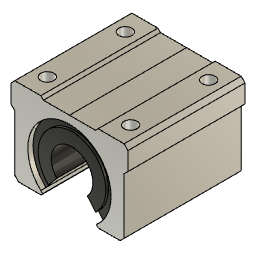
SBR16UU (Autodesk Fusion 360 design; units mm, degrees)
Autodesk Fusion 360 part; units mm, degrees
sketch "Front" plane through (0, 0, 0) normal (0, 1, 0) x (1, 0, 0)
  line L0 (-50, 19) -> (50, 19) construction
  line L1 (-50, 20) -> (50, 20) construction
  line L2 (-21, -21) -> (-21, 22) construction
  line L3 (21, -21) -> (21, 22) construction
  line L4 (-22.5, -21) -> (-22.5, 22) construction
  line L5 (22.5, -21) -> (22.5, 22) construction
  line L6 (-50, 10) -> (50, 10) construction
  line L7 (-10, 22) -> (-10, 0) construction
  line L8 (10, 22) -> (10, 0) construction
  line L9 (-11, 17) -> (-11, 22) construction
  line L10 (11, 17) -> (11, 22) construction
  line L11 (0, 19) -> (10, 19)
  line L12 (10, 19) -> (11, 20)
  line L13 (11, 20) -> (21, 20)
  line L14 (-50, 18.5) -> (50, 18.5) construction
  line L15 (21, 20) -> (22.5, 18.5)
  line L16 (-50, 11.5) -> (44, 11.5) construction
  line L17 (22.5, 18.5) -> (22.5, 11.5)
  line L18 (22.5, 11.5) -> (21, 10)
  line L19 (-24, -19) -> (25, -19) construction
  line L20 (-25, -11.5) -> (25, -11.5) construction
  line L21 (21, 10) -> (21, -11.5)
  line L22 (19.5, -15) -> (19.5, -9) construction
  line L23 (-19.5, -15) -> (-19.5, -10) construction
  line L24 (21, -11.5) -> (19.5, -13)
  line L25 (-19.5, -13) -> (-21, -11.5)
  line L26 (-21, -11.5) -> (-21, 10)
  line L27 (-21, 10) -> (-22.5, 11.5)
  line L28 (-22.5, 11.5) -> (-22.5, 18.5)
  line L29 (-22.5, 18.5) -> (-21, 20)
  line L30 (-21, 20) -> (-11, 20)
  line L31 (-11, 20) -> (-10, 19)
  line L32 (-10, 19) -> (0, 19)
  line L33 (5.1423, -6.1284) -> (10.9083, -13)
  line L34 (-5.1423, -6.1284) -> (-10.9083, -13)
  line L35 (0, 0) -> (18.416, 0) construction
  line L36 (0, -18) -> (0, -16)
  arc A0 (10.2846, -12.2567) -> (-10.2846, -12.2567) centre (0, 0) ccw
  line L37 (-10.9083, -13) -> (-19.5, -13)
  line L38 (-50, -13) -> (-10.9083, -13) construction
  line L39 (-0.0022, -13) -> (44, -13) construction
  line L40 (19.5, -13) -> (10.9083, -13)
  line L41 (0.0022, -13) -> (-0.0022, -13)
  arc A1 (8.3562, -9.9586) -> (-8.3562, -9.9586) centre (0, 0) ccw
  arc A2 (-0.0022, -13) -> (0.0022, -13) centre (0, 0) ccw
  arc A3 (5.1423, -6.1284) -> (-5.1423, -6.1284) centre (0, 0) ccw
  dimension "d3" = 1
  dimension "d4" = 19
  dimension "d5" = 13
  dimension "d7" = 21
  dimension "d8" = 1.5
  dimension "d9" = 1.5
  dimension "d10" = 10
  dimension "d11" = 10
  dimension "d13" = 10
  dimension "d14" = 1
  dimension "d15" = 1
  dimension "d16" = 0.5
  dimension "d17" = 1.5
  dimension "d19" = 1.5
  dimension "d20" = 1.5
  dimension "d21" = 1.5
  dimension "d23" = 130
  constraint coincident L35.start A0.centre
  constraint concentric A1 A3
  constraint concentric A0 A1
  constraint horizontal L0
  constraint horizontal L1
  constraint horizontal L38
  constraint perpendicular L1 L2
  constraint perpendicular L1 L3
  constraint perpendicular L1 L4
  constraint perpendicular L1 L5
  constraint perpendicular L4 L6
  constraint perpendicular L6 L7
  constraint perpendicular L6 L8
  constraint perpendicular L1 L9
  constraint perpendicular L1 L10
  constraint midpoint L0 L11.start
  constraint coincident L8 L11.end
  constraint coincident L0 L11.end
  constraint coincident L1 L12.end
  constraint coincident L10 L12.end
  constraint coincident L3 L13.end
  constraint coincident L1 L13.end
  constraint perpendicular L5 L14
  constraint coincident L5 L15.end
  constraint coincident L14 L15.end
  constraint parallel L6 L16
  constraint coincident L5 L17.end
  constraint coincident L16 L17.end
  constraint coincident L3 L18.end
  constraint perpendicular L5 L19
  constraint perpendicular L5 L20
  constraint coincident L3 L21.end
  constraint coincident L20 L21.end
  constraint perpendicular L20 L21
  constraint perpendicular L20 L22
  constraint perpendicular L20 L23
  constraint coincident L24.end L38
  constraint coincident L22 L24.end
  constraint coincident L25.start L38
  constraint coincident L23 L25.start
  constraint coincident L20 L25.end
  constraint coincident L2 L25.end
  constraint coincident L6 L26.end
  constraint coincident L2 L26.end
  constraint coincident L4 L27.end
  constraint coincident L16 L27.end
  constraint coincident L4 L28.end
  constraint coincident L14 L28.end
  constraint coincident L2 L29.end
  constraint coincident L1 L29.end
  constraint coincident L1 L30.end
  constraint coincident L9 L30.end
  constraint coincident L0 L31.end
  constraint coincident L7 L31.end
  constraint horizontal L35
  constraint collinear L37 L40
  constraint coincident L34 A0.end
  constraint coincident L39.start A1
  constraint collinear L38 L39
  constraint collinear L40 L41
  constraint coincident L39 L41.start
  constraint coincident L33 A1.start
  constraint coincident L33 A0.start
  constraint coincident L34 A1.end
  constraint concentric A1 A2
  measures "d3" distance of L0 L1
  measures "d4" distance of L35.start L0
  measures "d5" distance of L35.start L38
  measures "d7" distance of L35.start L3
  measures "d8" distance of L2 L4
  measures "d9" distance of L3 L5
  measures "d10" distance of L1 L6
  measures "d11" distance of L35.start L7
  measures "d13" distance of L35.start L8
  measures "d14" distance of L7 L9
  measures "d15" distance of L8 L10
  measures "d16" distance of L0 L14
  measures "d17" distance of L6 L16
  measures "d19" distance of L20 L38
  measures "d20" distance of L2 L23
  measures "d21" distance of L3 L22
  measures "d23" angle of L34 L35
extrude "Extrude1" add sketch "Front" along normal blind 45 contours L11 L12 L13 L15 L17 L18 L21 L24 L25 L26 L27 L28 L29 L30 L31 L32 L33 L34 A0 L37 L40 makes body 1
extrude "Extrude2" add sketch "Front" along normal blind 38 contours L33 L34 A0 A1 bodies 1
extrude "Extrude3" cut sketch "Front" along normal blind 2 contours L33 L34 A0 A1 bodies 1
extrude "Extrude4" add 1 faces at (-10.2071, 38, 10.9401) along direction (0, 1, 0) blind 5 on bodies 1 bodies 1
extrude "Extrude5" add sketch "Front" along normal blind 44 contours L33 L34 A1 A3 bodies 1
extrude "Extrude6" cut sketch "Front" along normal blind 1 contours L33 L34 A1 A3 bodies 1
sketch "Sketch4" plane through (0, 0, 0) normal (0.766044, 0, 0.642788) x (0, 1, 0)
  line L0 (1, 13) -> (1, 8)
  line L1 (1, 8) -> (44, 8)
  line L2 (44, 8) -> (44, 13)
  line L3 (44, 13) -> (43, 13)
  line L4 (43, 13) -> (43, 16)
  line L5 (43, 16) -> (45, 16)
  line L6 (45, 16) -> (45, 16.9703)
  line L7 (45, 16.9703) -> (0, 16.9703)
  line L8 (0, 16.9703) -> (0, 16)
  line L9 (0, 16) -> (2, 16)
  line L10 (2, 16) -> (2, 13)
  line L11 (2, 13) -> (1, 13)
  line L12 (2, 16) -> (43, 16) construction
  line L13 (22.5, 16) -> (46, 16)
  line L14 (46, 16) -> (46, 7)
  line L15 (46, 7) -> (22.5, 7)
  line L16 (22.5, 7) -> (22.5, 16)
  line L17 (22.5, 16) -> (-1, 16)
  line L18 (-1, 16) -> (-1, 7)
  line L19 (-1, 7) -> (22.5, 7)
  line L20 (22.5, 7) -> (22.5, 16)
  constraint coincident L9.end L10.start
  constraint coincident L4.end L5.start
  constraint horizontal L13
  constraint vertical L14
  constraint horizontal L15
  constraint vertical L16
  constraint midpoint L12 L13.start
  constraint horizontal L17
  constraint vertical L18
  constraint horizontal L19
  constraint vertical L20
extrude "Extrude7" cut sketch "Sketch4" against normal blind 1 contours L0 L1 L10 L11 L16 L17 L20 | L0 L1 L9 L10 L11 L16 L17 L18 L19 L20 | L1 L2 L3 L4 L13 L16 L20 | L1 L2 L3 L4 L5 L13 L14 L15 L16 L20 bodies 1
sketch "Sketch5" plane through (0, 0, 0) normal (-0.766044, 0, 0.642788) x (0, -1, 0)
  line L0 (-1, 8) -> (-1, 13)
  line L1 (-1, 13) -> (-2, 13)
  line L2 (-2, 13) -> (-2, 16)
  line L3 (-2, 16) -> (0, 16)
  line L4 (0, 16) -> (0, 16.9703)
  line L5 (0, 16.9703) -> (-45, 16.9703)
  line L6 (-45, 16.9703) -> (-45, 16)
  line L7 (-45, 16) -> (-43, 16)
  line L8 (-43, 16) -> (-43, 13)
  line L9 (-43, 13) -> (-44, 13)
  line L10 (-44, 13) -> (-44, 8)
  line L11 (-44, 8) -> (-1, 8)
  line L12 (-43, 16) -> (-2, 16)
  line L13 (-22.5, 16) -> (1, 16)
  line L14 (1, 16) -> (1, 7)
  line L15 (1, 7) -> (-22.5, 7)
  line L16 (-22.5, 7) -> (-22.5, 16)
  line L17 (-22.5, 16) -> (-46, 16)
  line L18 (-46, 16) -> (-46, 7)
  line L19 (-46, 7) -> (-22.5, 7)
  line L20 (-22.5, 7) -> (-22.5, 16)
  constraint coincident L7.end L8.start
  constraint coincident L2.end L3.start
  constraint horizontal L13
  constraint vertical L14
  constraint horizontal L15
  constraint vertical L16
  constraint midpoint L12 L13.start
  constraint horizontal L17
  constraint vertical L18
  constraint horizontal L19
  constraint vertical L20
extrude "Extrude8" cut sketch "Sketch5" against normal blind 1 contours L0 L1 L2 L11 L12 L13 L16 L20 | L0 L1 L2 L3 L11 L13 L14 L15 L16 L20 | L7 L8 L9 L10 L11 L16 L17 L18 L19 L20 | L8 L9 L10 L11 L12 L16 L17 L20 bodies 1
move_body "Move1" bodies 1 to x (-1, 0, 0) y (0, 1, 0) z (0, 0, -1) at (0, 0, 0)
sketch "Top" plane through (0, 0, 20) normal (0, 0, 1) x (-1, 0, 0)
  line L0 (21, 0) -> (11, 0)
  line L1 (11, 0) -> (11, -45)
  line L2 (11, -45) -> (21, -45)
  line L3 (21, -45) -> (21, 0)
  line L4 (16, -37.5) -> (-16, -37.5) construction
  line L5 (-16, -37.5) -> (-16, -7.5) construction
  line L6 (-16, -7.5) -> (16, -7.5) construction
  line L7 (16, -7.5) -> (16, -37.5) construction
  line L8 (-10, 0) -> (0, 0) construction
  line L9 (0, 0) -> (0, -45) construction
  circle A0 centre (16, -37.5) radius 2.5
  circle A1 centre (-16, -37.5) radius 2.5
  circle A2 centre (-16, -7.5) radius 2.5
  circle A3 centre (16, -7.5) radius 2.5
  dimension "d41" = 32
  dimension "d42" = 30
  dimension "d43" = 7.5
  dimension "d44" = 16
  dimension "d45" = 5
  dimension "d46" = 5
  dimension "d47" = 5
  dimension "d48" = 5
  constraint horizontal L4
  constraint vertical L5
  constraint horizontal L6
  constraint vertical L7
  constraint coincident L4.start L7.end
  constraint coincident L4.end L5.start
  constraint coincident L5.end L6.start
  constraint coincident L6.end L7.start
  measures "d41" distance of L4.start L4.end
  measures "d42" distance of L4.start L6.end
  measures "d43" distance of L6 L8
  measures "d44" distance of L5 L9
  measures "d45" diameter of A0
  measures "d46" diameter of A1
  measures "d47" diameter of A2
  measures "d48" diameter of A3
extrude "Extrude9" cut sketch "Top" against normal blind 12 contours A0 | A1 | A2 | A3 bodies 1
copy_body "Body->Comp1" bodies 1 removing the originals makes body 2 in component "SBR16UU"
component "SBR16UU" placed x (1, 0, 0) y (0, 1, 0) z (0, 0, 1) at (0, 0, 0)
named bodies: "SBR16UU"
